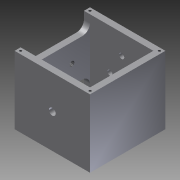
# Autodesk Inventor part: 1_0204_001
Saved by Autodesk Inventor 2012 SP1 (Build 160190100, 190)
## iProperties
Created: 2013-03-22
Part Number: 1_0204_001
Material: Default
Document SubType Name: Modeling
Designer: vogel
Density: 1 g/cm^3
Author: vogel
Autodesk Inventor part; units mm, degrees
note: some values were not read from the file. Chosen so that the rebuilt part matches the saved one: direction of "Bohrung1"; direction of "Bohrung2".
ref_plane "YZ Plane" through (0, 0, 0) normal (1, 0, 0) x (0, 1, 0)
ref_plane "XZ Plane" through (0, 0, 0) normal (0, 1, 0) x (-1, 0, 0)
sketch "Skizze1" plane through (0, 0, 0) normal (0, 0, 1) x (1, 0, 0)
  line L0 (-25, 25) -> (25, 25)
  line L1 (25, 25) -> (25, -25)
  line L2 (25, -25) -> (-25, -25)
  line L3 (-25, -25) -> (-25, 25)
  line L4 (-35, 0) -> (35, 0) projected
  line L5 (0, -35) -> (0, 35) projected
  line L6 (21, 21) -> (-21, 21)
  line L7 (-21, 21) -> (-21, -21)
  line L8 (-21, -21) -> (21, -21)
  line L9 (21, -21) -> (21, 21)
  point P0 (0, 0)
  dimension "d0" = 50
  dimension "d1" = 50
  dimension "d2" = 4
  constraints: 16 end point, 4 parallel, 2 perpendicular, 1 horizontal, 5 other
  measures "d0" distance between parallel lines of L2 L0
  measures "d1" distance between parallel lines of L1 L3
  measures "d2" distance between parallel lines of L0 L6
extrude "Extrusion1" add sketch "Skizze1" along normal blind 45 contours L0 L5 L6 L7 L4 L3 | L0 L1 L4 L9 L6 L5 | L4 L7 L8 L5 L2 L3 | L1 L2 L5 L8 L9 L4
sketch "Skizze2" plane through (-25, -25, 0) normal (-1, 0, 0) x (0, 0, 1)
  line L0 (0, 50) -> (45, 50) projected
  line L1 (0, 0) -> (45, 0) projected
  line L2 (22.5, 50) -> (22.5, 0)
  line L3 (0, 46) -> (45, 46) projected
  line L4 (0, 4) -> (45, 4) projected
  line L5 (0, 46) -> (5, 46)
  line L6 (10, 41) -> (10, 9)
  line L7 (5, 4) -> (0, 4)
  line L8 (0, 4) -> (0, 46)
  line L9 (45, 4) -> (40, 4)
  line L10 (35, 9) -> (35, 41)
  line L11 (40, 46) -> (45, 46)
  line L12 (45, 46) -> (45, 4)
  arc A0 (40, 46) -> (35, 41) centre (40, 41) ccw
  arc A1 (35, 9) -> (40, 4) centre (40, 9) ccw
  arc A2 (5, 4) -> (10, 9) centre (5, 9) ccw
  arc A3 (10, 41) -> (5, 46) centre (5, 41) ccw
  point P0 (0, 25)
  point P1 (10, 4)
  point P2 (35, 46)
  dimension "d5" = 25
  dimension "d6" = 5
  constraints: 18 end point, 8 point on circle, 8 tangent, 6 point on line, 4 centre point, 4 parallel, 3 equal radius, 2 horizontal, 2 midpoint, 2 perpendicular, 1 other
  measures "d5" distance between parallel lines of L6 L10
  measures "d6" radius of A0
extrude "Extrusion2" cut sketch "Skizze2" against normal up to surface (46 mm away) contours A3 L6 A2 L4 L8 L3 | L3 L12 L4 A1 L10 A0
sketch "Skizze3" plane through (-25, 25, 0) normal (0, 1, 0) x (1, 0, 0)
  line L0 (0, -45) -> (50, -45) projected
  line L1 (50, 0) -> (50, -45) projected
  line L2 (0, 0) -> (0, -45) projected
  line L3 (50, -22.5) -> (0, -22.5)
  line L4 (25, -45) -> (25, 0)
  circle A0 centre (25, -22.5) radius 9
  line L5 (25, -22.5) -> (17.2058, -18)
  line L6 (25, -22.5) -> (32.7942, -18)
  point P0 (25, -31.5)
  dimension "d9" = 18
  dimension "d10" = 120
  dimension "d11" = 120
  constraints: 8 end point, 4 midpoint, 3 point on circle, 1 centre point, 1 perpendicular, 1 point on line
  measures "d9" diameter of A0
  measures "d10" angle of L5 L4
  measures "d11" angle of L6 L4
hole "Bohrung1" at (0, 25, 31.5) at (-7.7942, 25, 18) at (7.7942, 25, 18) direction (0, -1, 0) diameter 3.4 end up to surface countersink diameter 6.9 countersink angle 90
sketch "Skizze4" plane through (-25, -25, 0) normal (0, -1, 0) x (1, 0, 0)
  line L0 (50, 45) -> (0, 45) projected
  line L1 (0, 0) -> (0, 45) projected
  line L2 (50, 0) -> (50, 45) projected
  line L3 (0, 22.5) -> (50, 22.5)
  line L4 (25, 45) -> (25, 0)
  circle A0 centre (25, 22.5) radius 2.25
  dimension "d19" = 4.5
  constraints: 4 end point, 4 midpoint, 1 centre point, 1 perpendicular
  measures "d19" diameter of A0
extrude "Extrusion3" cut sketch "Skizze4" against normal up to surface (46 mm away) contours A0 L3 L4 | L4 L3 A0 | A0 L4 L3 | L4 A0 L3
sketch "Skizze5" plane through (-25, 21, 0) normal (-1, 0, 0) x (0, 0, 1)
  circle A0 centre (22.5, -30) radius 2.25 projected
  circle A1 centre (22.5, -12) radius 2.25 projected
  line L0 (35, -35) -> (35, -6) projected
  line L1 (10, -6) -> (35, -6) projected
  line L2 (10, -6) -> (10, -35) projected
  arc A2 (5, -40) -> (10, -35) centre (5, -35) ccw projected
  line L3 (5, -40) -> (40, -40) projected
  arc A3 (35, -35) -> (40, -40) centre (40, -35) ccw projected
  point P0 (0, -21)
  constraints: 2 coincident
hole "Bohrung2" at (-25, 9, 22.5) at (-25, -9, 22.5) direction (1, 0, 0) diameter 3.242 end up to surface thread size "M4x0.7" class "6H" standard "ISO Metric profile"
sketch "Skizze6" plane through (0, 0, 45) normal (0, 0, 1) x (1, 0, 0)
  line L0 (-25, -25) -> (-25, -21) projected
  line L1 (25, -25) -> (-25, -25) projected
  line L2 (25, 25) -> (25, -25) projected
  line L3 (-25, 25) -> (25, 25) projected
  line L4 (-25, 21) -> (-25, 25) projected
  line L5 (-25, 23) -> (25, 23)
  line L6 (23, 25) -> (23, -25)
  line L7 (-25, -23) -> (25, -23)
  line L8 (-23, 25) -> (-23, -25)
  point P0 (0, 0)
  point P1 (-23, 23)
  point P2 (23, 23)
  point P3 (23, -23)
  point P4 (-23, -23)
  dimension "d29" = 2
  dimension "d30" = 2
  constraints: 14 point on line, 8 end point, 4 perpendicular, 2 midpoint
  measures "d29" distance between parallel lines of L6 L2
  measures "d30" distance between parallel lines of L4 L8
hole "Bohrung3" at (-23, 23, 45) at (23, 23, 45) at (23, -23, 45) at (-23, -23, 45) direction (0, 0, -1) diameter 1.567 depth 8 tip angle 118 thread size "M2x0.4" class "6H" standard "ISO Metric profile"
ref_plane "Arbeitsebene1" through (0, 0, 22.5) normal (0, 0, 1) x (1, 0, 0)
mirror "Spiegeln1" about plane through (0, 0, 22.5) normal (0, 0, 1) of "Bohrung3"
